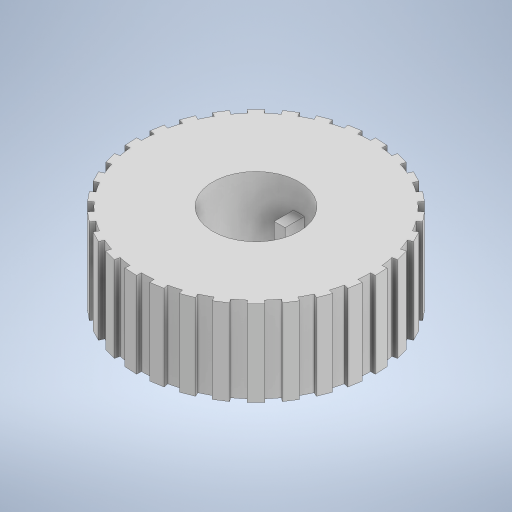
# Autodesk Inventor part: DialKnob
Saved by Autodesk Inventor 2024 (Build 280153000, 153)
## iProperties
Created: 2023-11-18
Part Number: DialKnob
Material: Generic
Document SubType Name: Modeling
Designer: gcter
Density: 1 g/cm^3
Appearance: Default
Author: gcter
Autodesk Inventor part; units mm, degrees
ref_plane "YZ Plane" through (0, 0, 0) normal (1, 0, 0) x (0, 1, 0)
ref_plane "XZ Plane" through (0, 0, 0) normal (0, 1, 0) x (-1, 0, 0)
ref_plane "XY Plane" through (0, 0, 0) normal (0, 0, 1) x (1, 0, 0)
sketch "Sketch1" plane through (0, 0, 0) normal (0, 1, 0) x (-1, 0, 0)
  arc A0 (-1.6643, -7.826) -> (-0.8372, -7.9571) centre (0, 0) ccw
  line L0 (-0.0008, -8.0004) -> (-0.0009, -8.3312)
  line L1 (-0.8372, -7.9571) -> (-0.8717, -8.2855)
  circle A1 centre (0, 0) radius 8.3312 construction
  line L2 (-0.0009, -8.3312) -> (-0.8717, -8.2855)
  line L3 (-1.6643, -7.826) -> (-1.733, -8.149) construction
  line L4 (1.6626, -7.8258) -> (1.7313, -8.1493)
  line L5 (1.7313, -8.1493) -> (0.87, -8.2857)
  line L6 (0.8355, -7.9573) -> (0.87, -8.2857)
  arc A2 (-0.0008, -8.001) -> (0.8355, -7.9573) centre (0, 0) ccw
  line L7 (3.2533, -7.3091) -> (3.3878, -7.6113)
  line L8 (3.3878, -7.6113) -> (2.5737, -7.9237)
  line L9 (2.4717, -7.6097) -> (2.5737, -7.9237)
  arc A3 (1.6627, -7.8263) -> (2.4717, -7.6097) centre (0, 0) ccw
  line L10 (4.7019, -6.473) -> (4.8963, -6.7406)
  line L11 (4.8963, -6.7406) -> (4.1649, -7.2155)
  line L12 (3.9998, -6.9295) -> (4.1649, -7.2155)
  arc A4 (3.2535, -7.3096) -> (3.9998, -6.9295) centre (0, 0) ccw
  line L13 (5.9449, -5.3539) -> (6.1907, -5.5753)
  line L14 (6.1907, -5.5753) -> (5.574, -6.1919)
  line L15 (5.3531, -5.9465) -> (5.574, -6.1919)
  arc A5 (4.7022, -6.4734) -> (5.3531, -5.9465) centre (0, 0) ccw
  line L16 (6.9282, -4.0009) -> (7.2146, -4.1663)
  line L17 (7.2146, -4.1663) -> (6.7396, -4.8977)
  line L18 (6.4725, -4.7035) -> (6.7396, -4.8977)
  arc A6 (5.9453, -5.3543) -> (6.4725, -4.7035) centre (0, 0) ccw
  line L19 (7.6086, -2.4731) -> (7.9232, -2.5753)
  line L20 (7.9232, -2.5753) -> (7.6106, -3.3894)
  line L21 (7.3089, -3.2551) -> (7.6106, -3.3894)
  arc A7 (6.9287, -4.0012) -> (7.3089, -3.2551) centre (0, 0) ccw
  line L22 (7.9565, -0.8371) -> (8.2855, -0.8717)
  line L23 (8.2855, -0.8717) -> (8.149, -1.733)
  line L24 (7.826, -1.6643) -> (8.149, -1.733)
  arc A8 (7.6091, -2.4732) -> (7.826, -1.6643) centre (0, 0) ccw
  line L25 (7.9567, 0.8354) -> (8.2857, 0.87)
  line L26 (8.2857, 0.87) -> (8.3312, -0.0009)
  line L27 (8.001, -0.0008) -> (8.3312, -0.0009)
  arc A9 (7.9571, -0.8372) -> (8.001, -0.0008) centre (0, 0) ccw
  line L28 (7.6091, 2.4715) -> (7.9237, 2.5737)
  line L29 (7.9237, 2.5737) -> (8.1493, 1.7313)
  line L30 (7.8263, 1.6627) -> (8.1493, 1.7313)
  arc A10 (7.9573, 0.8355) -> (7.8263, 1.6627) centre (0, 0) ccw
  line L31 (6.929, 3.9995) -> (7.2155, 4.1649)
  line L32 (7.2155, 4.1649) -> (7.6113, 3.3878)
  line L33 (7.3096, 3.2535) -> (7.6113, 3.3878)
  arc A11 (7.6097, 2.4717) -> (7.3096, 3.2535) centre (0, 0) ccw
  line L34 (5.946, 5.3527) -> (6.1919, 5.574)
  line L35 (6.1919, 5.574) -> (6.7406, 4.8963)
  line L36 (6.4734, 4.7022) -> (6.7406, 4.8963)
  arc A12 (6.9295, 3.9998) -> (6.4734, 4.7022) centre (0, 0) ccw
  line L37 (4.7032, 6.472) -> (4.8977, 6.7396)
  line L38 (4.8977, 6.7396) -> (5.5753, 6.1907)
  line L39 (5.3543, 5.9453) -> (5.5753, 6.1907)
  arc A13 (5.9465, 5.3531) -> (5.3543, 5.9453) centre (0, 0) ccw
  line L40 (3.2548, 7.3084) -> (3.3894, 7.6106)
  line L41 (3.3894, 7.6106) -> (4.1663, 7.2146)
  line L42 (4.0012, 6.9287) -> (4.1663, 7.2146)
  arc A14 (4.7035, 6.4725) -> (4.0012, 6.9287) centre (0, 0) ccw
  line L43 (1.6642, 7.8254) -> (1.733, 8.149)
  line L44 (1.733, 8.149) -> (2.5753, 7.9232)
  line L45 (2.4732, 7.6091) -> (2.5753, 7.9232)
  arc A15 (3.2551, 7.3089) -> (2.4732, 7.6091) centre (0, 0) ccw
  line L46 (0.0008, 8.0004) -> (0.0009, 8.3312)
  line L47 (0.0009, 8.3312) -> (0.8717, 8.2855)
  line L48 (0.8372, 7.9571) -> (0.8717, 8.2855)
  arc A16 (1.6643, 7.826) -> (0.8372, 7.9571) centre (0, 0) ccw
  line L49 (-1.6626, 7.8258) -> (-1.7313, 8.1493)
  line L50 (-1.7313, 8.1493) -> (-0.87, 8.2857)
  line L51 (-0.8355, 7.9573) -> (-0.87, 8.2857)
  arc A17 (0.0008, 8.001) -> (-0.8355, 7.9573) centre (0, 0) ccw
  line L52 (-3.2533, 7.3091) -> (-3.3878, 7.6113)
  line L53 (-3.3878, 7.6113) -> (-2.5737, 7.9237)
  line L54 (-2.4717, 7.6097) -> (-2.5737, 7.9237)
  arc A18 (-1.6627, 7.8263) -> (-2.4717, 7.6097) centre (0, 0) ccw
  line L55 (-4.7019, 6.473) -> (-4.8963, 6.7406)
  line L56 (-4.8963, 6.7406) -> (-4.1649, 7.2155)
  line L57 (-3.9998, 6.9295) -> (-4.1649, 7.2155)
  arc A19 (-3.2535, 7.3096) -> (-3.9998, 6.9295) centre (0, 0) ccw
  line L58 (-5.9449, 5.3539) -> (-6.1907, 5.5753)
  line L59 (-6.1907, 5.5753) -> (-5.574, 6.1919)
  line L60 (-5.3531, 5.9465) -> (-5.574, 6.1919)
  arc A20 (-4.7022, 6.4734) -> (-5.3531, 5.9465) centre (0, 0) ccw
  line L61 (-6.9282, 4.0009) -> (-7.2146, 4.1663)
  line L62 (-7.2146, 4.1663) -> (-6.7396, 4.8977)
  line L63 (-6.4725, 4.7035) -> (-6.7396, 4.8977)
  arc A21 (-5.9453, 5.3543) -> (-6.4725, 4.7035) centre (0, 0) ccw
  line L64 (-7.6086, 2.4731) -> (-7.9232, 2.5753)
  line L65 (-7.9232, 2.5753) -> (-7.6106, 3.3894)
  line L66 (-7.3089, 3.2551) -> (-7.6106, 3.3894)
  arc A22 (-6.9287, 4.0012) -> (-7.3089, 3.2551) centre (0, 0) ccw
  line L67 (-7.9565, 0.8371) -> (-8.2855, 0.8717)
  line L68 (-8.2855, 0.8717) -> (-8.149, 1.733)
  line L69 (-7.826, 1.6643) -> (-8.149, 1.733)
  arc A23 (-7.6091, 2.4732) -> (-7.826, 1.6643) centre (0, 0) ccw
  line L70 (-7.9567, -0.8354) -> (-8.2857, -0.87)
  line L71 (-8.2857, -0.87) -> (-8.3312, 0.0009)
  line L72 (-8.001, 0.0008) -> (-8.3312, 0.0009)
  arc A24 (-7.9571, 0.8372) -> (-8.001, 0.0008) centre (0, 0) ccw
  line L73 (-7.6091, -2.4715) -> (-7.9237, -2.5737)
  line L74 (-7.9237, -2.5737) -> (-8.1493, -1.7313)
  line L75 (-7.8263, -1.6627) -> (-8.1493, -1.7313)
  arc A25 (-7.9573, -0.8355) -> (-7.8263, -1.6627) centre (0, 0) ccw
  line L76 (-6.929, -3.9995) -> (-7.2155, -4.1649)
  line L77 (-7.2155, -4.1649) -> (-7.6113, -3.3878)
  line L78 (-7.3096, -3.2535) -> (-7.6113, -3.3878)
  arc A26 (-7.6097, -2.4717) -> (-7.3096, -3.2535) centre (0, 0) ccw
  line L79 (-5.946, -5.3527) -> (-6.1919, -5.574)
  line L80 (-6.1919, -5.574) -> (-6.7406, -4.8963)
  line L81 (-6.4734, -4.7022) -> (-6.7406, -4.8963)
  arc A27 (-6.9295, -3.9998) -> (-6.4734, -4.7022) centre (0, 0) ccw
  line L82 (-4.7032, -6.472) -> (-4.8977, -6.7396)
  line L83 (-4.8977, -6.7396) -> (-5.5753, -6.1907)
  line L84 (-5.3543, -5.9453) -> (-5.5753, -6.1907)
  arc A28 (-5.9465, -5.3531) -> (-5.3543, -5.9453) centre (0, 0) ccw
  line L85 (-3.2548, -7.3084) -> (-3.3894, -7.6106)
  line L86 (-3.3894, -7.6106) -> (-4.1663, -7.2146)
  line L87 (-4.0012, -6.9287) -> (-4.1663, -7.2146)
  arc A29 (-4.7035, -6.4725) -> (-4.0012, -6.9287) centre (0, 0) ccw
  line L88 (-1.6642, -7.8254) -> (-1.733, -8.149)
  line L89 (-1.733, -8.149) -> (-2.5753, -7.9232)
  line L90 (-2.4732, -7.6091) -> (-2.5753, -7.9232)
  arc A30 (-3.2551, -7.3089) -> (-2.4732, -7.6091) centre (0, 0) ccw
  point P0 (-0.0008, -8.001)
  point P1 (1.6627, -7.8263)
  point P2 (3.2535, -7.3096)
  point P3 (4.7022, -6.4734)
  point P4 (5.9453, -5.3543)
  point P5 (6.9287, -4.0012)
  point P6 (7.6091, -2.4732)
  point P7 (7.9571, -0.8372)
  point P8 (7.9573, 0.8355)
  point P9 (7.6097, 2.4717)
  point P10 (6.9295, 3.9998)
  point P11 (5.9465, 5.3531)
  point P12 (4.7035, 6.4725)
  point P13 (3.2551, 7.3089)
  point P14 (1.6643, 7.826)
  point P15 (0.0008, 8.001)
  point P16 (-1.6627, 7.8263)
  point P17 (-3.2535, 7.3096)
  point P18 (-4.7022, 6.4734)
  point P19 (-5.9453, 5.3543)
  point P20 (-6.9287, 4.0012)
  point P21 (-7.6091, 2.4732)
  point P22 (-7.9571, 0.8372)
  point P23 (-7.9573, -0.8355)
  point P24 (-7.6097, -2.4717)
  point P25 (-6.9295, -3.9998)
  point P26 (-5.9465, -5.3531)
  point P27 (-4.7035, -6.4725)
  point P28 (-3.2551, -7.3089)
  point P29 (-1.6643, -7.826)
  dimension "d0" = 16.002
  dimension "d1" = 6
  dimension "d2" = 0.3302
  dimension "d3" = 6
  dimension "d6" = 360
  constraints: 182 end point, 63 point on circle, 31 centre point, 3 line through centre, 2 coincident, 301 other
  measures "d0" diameter of A0
  measures "d1" angle of L1 L0
  measures "d2" radial gap between concentric circles of A0 A1
  measures "d3" angle of L1 L3
extrude "Extrusion1" add sketch "Sketch1" along normal blind 5.969
sketch "Sketch2" plane through (0, 5.969, 0) normal (0, 1, 0) x (1, 0, 0)
  arc A0 (-0.381, 2.9857) -> (0.381, 2.9857) centre (0, 0) ccw
  line L0 (0, 3.0099) -> (0, -3.0099) construction
  line L1 (-0.381, 1.651) -> (0.381, 1.651)
  line L2 (-0.381, 1.651) -> (-0.381, 2.9857)
  line L3 (0.381, 1.651) -> (0.381, 2.9857)
  dimension "d10" = 6.0198
  dimension "d13" = 0.381
  dimension "d14" = 0.381
  dimension "d16" = 1.651
  constraints: 8 end point, 3 point on circle, 2 coincident, 2 vertical, 1 centre point, 1 horizontal, 1 midpoint, 1 parallel
  measures "d10" diameter of A0
  measures "d13" distance from line of L1.end L0
  measures "d14" distance from line of L0 L1.start
  measures "d16" distance from line of point (0, 0) L1
extrude "Extrusion2" cut sketch "Sketch2" against normal blind 4.699
sketch "Sketch3" plane through (0, 5.969, 0) normal (0, 1, 0) x (1, 0, 0)
  circle A0 centre (0, 0) radius 3.0099
  arc A1 (-0.381, 2.9857) -> (0.381, 2.9857) centre (0, 0) ccw projected
  constraints: 1 centre point, 1 coincident, 1 concentric
extrude "Extrusion3" cut sketch "Sketch3" against normal blind 1.905
body "Solid1"
